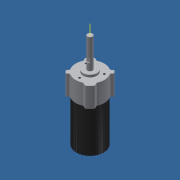
# Autodesk Inventor part: FaulhaberMotor
Saved by Autodesk Inventor 2014 SP2 (Build 180246200, 246)
## iProperties
Created: 2015-01-16
Part Number: FaulhaberMotor
Material: Aluminium 6061
Document SubType Name: Modeling
Designer: 4ndreas
Density: 2.71 g/cm^3
Appearance: Aluminium - flach
Author: 4ndreas
Autodesk Inventor part; units mm, degrees
ref_plane "YZ Plane" through (0, 0, 0) normal (1, 0, 0) x (0, 1, 0)
ref_plane "XZ Plane" through (0, 0, 0) normal (0, 1, 0) x (-1, 0, 0)
sketch "Skizze1" plane through (0, 0, 0) normal (0, 0, 1) x (1, 0, 0)
  circle A0 centre (0, 0) radius 8
  circle A1 centre (0, 0) radius 16.5
  arc A2 (-11.7062, 16.2162) -> (-16.2162, 11.7062) centre (0, 0) ccw
  arc A3 (-16.2162, 11.7062) -> (-16.3276, 10.13) centre (-15, 10.8282) ccw
  arc A4 (-15.1159, 6.6151) -> (-15.1625, 7.9147) centre (-16.4901, 7.2164) ccw
  line L0 (-16.3276, 10.13) -> (-15.1625, 7.9147)
  line L1 (-10.13, 16.3276) -> (-7.9147, 15.1625)
  arc A5 (-10.13, 16.3276) -> (-11.7062, 16.2162) centre (-10.8282, 15) ccw
  arc A6 (-7.9147, 15.1625) -> (-6.6151, 15.1159) centre (-7.2164, 16.4901) ccw
  arc A7 (-6.6151, 15.1159) -> (-15.1159, 6.6151) centre (0, 0) ccw
  line L2 (0, 0) -> (-16.2511, 16.2511) construction
  line L3 (0, 22.9833) -> (0, -21.5339) construction
  line L4 (-21.9209, 0) -> (29.1047, 0) construction
  line L5 (-16.5, 16.5) -> (16.5, 16.5) construction
  line L6 (16.5, 16.5) -> (16.5, -16.5) construction
  line L7 (16.5, -16.5) -> (-16.5, -16.5) construction
  line L8 (-16.5, -16.5) -> (-16.5, 16.5) construction
  line L9 (16.5, 16.5) -> (-16.5, -16.5) construction
  arc A8 (14.0181, 8.703) -> (8.703, 14.0181) centre (0, 0) ccw
  arc A9 (14.958, 13.2762) -> (13.2762, 14.958) centre (0, 0) ccw
  arc A10 (13.2762, 14.958) -> (11.2199, 14.8968) centre (12.2805, 13.8361) ccw
  arc A11 (8.703, 14.0181) -> (10.5549, 14.2318) centre (9.4942, 15.2925) ccw
  arc A12 (14.2318, 10.5549) -> (14.0181, 8.703) centre (15.2925, 9.4942) ccw
  arc A13 (14.8968, 11.2199) -> (14.958, 13.2762) centre (13.8361, 12.2805) ccw
  line L10 (11.2199, 14.8968) -> (10.5549, 14.2318)
  line L11 (14.2318, 10.5549) -> (14.8968, 11.2199)
  circle A14 centre (0, 0) radius 20 construction
  arc A15 (-14.0181, -8.703) -> (-8.703, -14.0181) centre (0, 0) ccw
  arc A16 (-14.958, -13.2762) -> (-13.2762, -14.958) centre (0, 0) ccw
  arc A17 (-14.8968, -11.2199) -> (-14.958, -13.2762) centre (-13.8361, -12.2805) ccw
  arc A18 (-14.2318, -10.5549) -> (-14.0181, -8.703) centre (-15.2925, -9.4942) ccw
  arc A19 (-8.703, -14.0181) -> (-10.5549, -14.2318) centre (-9.4942, -15.2925) ccw
  arc A20 (-13.2762, -14.958) -> (-11.2199, -14.8968) centre (-12.2805, -13.8361) ccw
  line L12 (-14.8968, -11.2199) -> (-14.2318, -10.5549)
  line L13 (-10.5549, -14.2318) -> (-11.2199, -14.8968)
  arc A21 (11.7062, -16.2162) -> (16.2162, -11.7062) centre (0, 0) ccw
  arc A22 (10.13, -16.3276) -> (11.7062, -16.2162) centre (10.8282, -15) ccw
  arc A23 (7.9147, -15.1625) -> (6.6151, -15.1159) centre (7.2164, -16.4901) ccw
  line L14 (10.13, -16.3276) -> (7.9147, -15.1625)
  line L15 (16.3276, -10.13) -> (15.1625, -7.9147)
  arc A24 (16.2162, -11.7062) -> (16.3276, -10.13) centre (15, -10.8282) ccw
  arc A25 (15.1159, -6.6151) -> (15.1625, -7.9147) centre (16.4901, -7.2164) ccw
  arc A26 (6.6151, -15.1159) -> (15.1159, -6.6151) centre (0, 0) ccw
  dimension "d0" = 33
  dimension "d1" = 16
  dimension "d2" = 45
  dimension "d3" = 1.5
  dimension "d4" = 10.25
  dimension "d5" = 40
  dimension "d6" = 5.2
  constraints: 48 point on circle, 32 end point, 27 centre point, 25 tangent, 24 symmetric about line, 9 coincident, 6 equal radius, 3 parallel, 2 perpendicular, 1 equal length, 1 horizontal, 1 vertical, 17 other
  measures "d0" diameter of A1
  measures "d1" diameter of A0
  measures "d2" angle of L4 L2
  measures "d3" radius of A5
  measures "d4" distance of L0.end L1.end
  measures "d5" diameter of A14
  measures "d6" distance between parallel lines of L11 L10
extrude "Extrusion1" add sketch "Skizze1" against normal blind 23 contours A0 | A1
extrude "Extrusion2" add sketch "Skizze1" against normal up to surface (23 mm away) contours A1 A11 L10 A10 A9 A13 L11 A12 | A25 L15 A24 A21 A22 L14 A23 A1 | A1 A4 L0 A3 A2 A5 L1 A6 | A19 L13 A20 A16 A17 L12 A18 A1
extrude "Extrusion3" add sketch "Skizze1" along normal blind 2.6 contours A0
sketch "Skizze2" plane through (0, 0, 2.6) normal (0, 0, 1) x (1, 0, 0)
  circle A0 centre (0, 0) radius 8 projected
  circle A1 centre (0, 0) radius 3
  dimension "d13" = 6
  constraints: 1 centre point, 1 coincident
  measures "d13" diameter of A1
extrude "Extrusion4" add sketch "Skizze2" along normal blind 34 contours A1
sketch "Skizze3" plane through (0, 0, -23) normal (0, 0, -1) x (-1, 0, 0)
  arc A0 (-13.2762, 14.958) -> (-14.958, 13.2762) centre (0, 0) ccw projected
  circle A1 centre (0, 0) radius 15.361
  constraints: 1 centre point, 1 coincident
extrude "Extrusion5" add sketch "Skizze3" along normal blind 50
sketch "Skizze4" plane through (0, 0, -73) normal (0, 0, -1) x (-1, 0, 0)
  circle A0 centre (0, 0) radius 15.361 projected
ref_plane "Arbeitsebene1" through (0, 0, 15.75) normal (0, 0, 1) x (1, 0, 0)
sketch "Skizze5" plane through (0, 0, 15.75) normal (0, 0, 1) x (1, 0, 0)
  circle A0 centre (0, 0) radius 3 projected
  line L0 (-2.08, 2.1619) -> (-2.08, -2.08)
  line L1 (-2.08, -2.08) -> (2.1619, -2.08)
  arc A1 (-2.08, 2.1619) -> (2.1619, -2.08) centre (0, 0) ccw
  dimension "d19" = 5.08
  dimension "d20" = 5.08
  constraints: 4 end point, 4 point on circle, 1 centre point, 1 coincident, 1 perpendicular, 1 vertical
extrude "Extrusion6" cut sketch "Skizze5" against normal blind 5.1 contours L0 L1 A0 picked at (0.5585, -2.2339)
sketch "Skizze6" plane through (0, 0, 0) normal (0, 0, 1) x (1, 0, 0)
  circle A0 centre (0, 0) radius 8 projected
  line L0 (-10.4, 6.0044) -> (0, -12.0089) construction
  line L1 (0, -12.0089) -> (10.4, 6.0044) construction
  line L2 (10.4, 6.0044) -> (-10.4, 6.0044) construction
  line L3 (10.4, 6.0044) -> (-5.2, -3.0022) construction
  line L4 (0, -12.0089) -> (0, 6.0044) construction
  dimension "d23" = 20.8
  constraints: 10 end point, 2 midpoint, 2 perpendicular, 2 point on line, 1 equal length, 1 horizontal
  measures "d23" distance of L1.end L0.start
hole "Bohrung1" at (-10.4, 6.0044, 0) at (10.4, 6.0044, 0) at (0, -12.0089, 0) direction (0, 0, -1) diameter 2.459 depth 8 tip angle 118 thread size "M3x0.5" class "6H" standard "ANSI Metric M Profile"
sketch "Skizze7" plane through (0, 0, -73) normal (0, 0, -1) x (-1, 0, 0)
  circle A0 centre (0, 0) radius 15.361 projected
  line L0 (-0.4, 15.961) -> (0.4, 15.961)
  line L1 (0.4, 15.961) -> (0.4, 14.761)
  line L2 (0.4, 14.761) -> (-0.4, 14.761)
  line L3 (-0.4, 14.761) -> (-0.4, 15.961)
  line L4 (0, -0.2243) -> (0, 15.361) construction
  dimension "d31" = 0.8
  dimension "d32" = 0.6
  dimension "d33" = 1.2
  constraints: 10 end point, 3 parallel, 1 horizontal, 1 perpendicular, 1 point on line, 1 vertical alignment, 2 other
  measures "d31" distance between parallel lines of L3 L1
  measures "d32" distance from line of L4.end L0
  measures "d33" distance between parallel lines of L0 L2
extrude "Extrusion7" add sketch "Skizze7" against normal up to surface (50 mm away) contours L1 L2 L3 A0 | A0 L3 L0 L1 picked at (0.0444, 14.9608)
pattern_circular "Runde Anordnung1" count 32 over 360 about axis through (0, 0, -23) along (0, 0, -1) of "Extrusion7"
equation "\"d20\" = d19"
equation "\"d33\" = 2 * d32"
